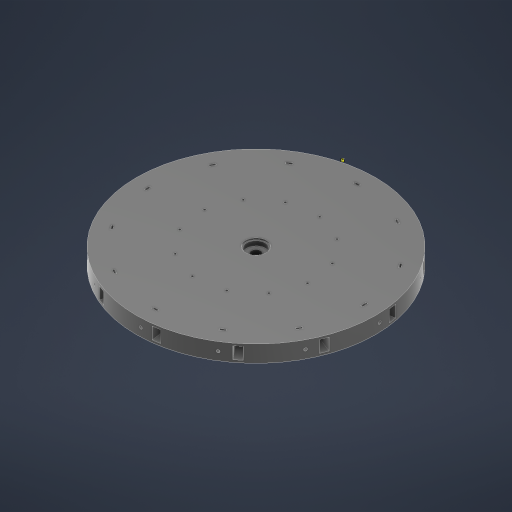
# Autodesk Inventor part: RotorBody
Saved by Autodesk Inventor 2023.1 (Build 271208000, 208)
## iProperties
Created: 2022-07-28
Part Number: RotorBody
Material: ABS Plastic
Document SubType Name: Modeling
Designer: ABL
Density: 1.06 g/cm^3
Appearance: Smooth - Black
Author: ABL
Autodesk Inventor part; units mm, degrees
ref_plane "YZ Plane" through (0, 0, 0) normal (1, 0, 0) x (0, 1, 0)
ref_plane "XZ Plane" through (0, 0, 0) normal (0, 1, 0) x (-1, 0, 0)
ref_plane "XY Plane" through (0, 0, 0) normal (0, 0, 1) x (1, 0, 0)
sketch "Sketch2" plane through (0, 0, 0) normal (0, 1, 0) x (-1, 0, 0)
  circle A0 centre (0, 0) radius 101.1611
  circle A1 centre (0, 0) radius 4.2
  dimension "d4" = 202.3223
  dimension "d101" = 8.4
  constraints: 2 centre point, 2 coincident
  measures "d4" diameter of A0
  measures "d101" diameter of A1
extrude "Extrusion1" add sketch "Sketch2" along normal blind 14.1
ref_plane "Work Plane4" through (-26.1824, 0, -97.7141) normal (-0.258819, 0, -0.9659258) x (0, -1, 0)
sketch "Sketch13" plane through (-27.2565, 0, -101.7227) normal (-0.258819, 0, -0.9659258) x (0, -1, 0)
  line L0 (-14.1, 101.1611) -> (-14.1, -101.1611) construction
  line L1 (0, 0) -> (-14.1, 0) construction
  line L2 (0, 0.05) -> (-14.1, 0.05)
  line L3 (-14.1, 0.05) -> (-14.1, -0.05)
  line L4 (-14.1, -0.05) -> (0, -0.05)
  line L5 (0, -0.05) -> (0, 0.05)
  line L6 (0, 0.05) -> (-14.1, -0.05) construction
  line L7 (-14.1, 0.05) -> (0, -0.05) construction
  point P0 (-7.05, 0)
  dimension "d136" = 0.1
  dimension "d139" = 7.05
  dimension "d140" = 2.05
  dimension "d141" = 4.2
  dimension "d142" = 3.8
  dimension "d146" = 4.1
  dimension "d147" = 4.3
  dimension "d153" = 4.2
  constraints: 8 end point, 2 parallel, 1 horizontal, 1 perpendicular
  measures "d153" distance of L2.end L3.end
sketch "Sketch10" plane through (0, 0, 0) normal (0, -1, 0) x (1, 0, 0)
  line L0 (0, 0) -> (-27.2565, -101.7227)
  line L1 (0, 0) -> (105.3111, 0) construction
  arc A0 (-27.2565, -101.7227) -> (30.0421, -100.9352) centre (0, 0) ccw
  line L2 (0, 0) -> (30.0421, -100.9352)
  line L3 (0, 0) -> (-27.2565, -101.7227) construction
  dimension "d96" = 105.3111
  dimension "d97" = 105
  dimension "d98" = 31.575
  constraints: 8 end point, 2 point on circle, 1 centre point, 1 coincident, 1 equal length, 1 horizontal
  measures "d96" distance of L0.start L0.end
  measures "d97" angle of L0 L1
  measures "d98" angle of L3 L2
sketch "Sketch8" plane through (0, 0, 0) normal (0, 1, 0) x (-1, 0, 0)
  circle A0 centre (0, 0) radius 105.3111
  circle A1 centre (0, 0) radius 101.2111
  circle A2 centre (0, 0) radius 4.2 projected
  line L0 (0, 0) -> (74.4662, -74.4662)
  line L1 (0, 0) -> (-101.7227, -27.2565)
  line L2 (0, 0) -> (0, -105.3111) construction
  point P0 (-97.7624, -26.1954)
  point P1 (71.5671, -71.5671)
  dimension "d81" = 210.6223
  dimension "d82" = 202.4223
  dimension "d184" = 120
  dimension "d185" = 45
  constraints: 6 end point, 3 point on circle, 2 centre point, 2 coincident, 1 vertical
  measures "d81" diameter of A0
  measures "d82" diameter of A1
  measures "d184" angle of L0 L1
  measures "d185" angle of L0 L2
extrude "Extrusion2" add sketch "Sketch8" along normal blind 14.1 separate body contours L1 A1 L0 A0 picked at (-26.5065, -98.9237)
pattern_circular "Circular Pattern5" [suppressed]
sketch "Sketch1" plane through (0, 0, 0) normal (0, 1, 0) x (-1, 0, 0)
  circle A0 centre (0, 0) radius 38.9611 construction
  arc A1 (-26.1824, -97.7141) -> (26.1824, -97.7141) centre (0, 0) ccw
  line L0 (0, 0) -> (26.1824, -97.7141)
  line L1 (0, 0) -> (101.1611, 0) construction
  line L2 (0, 0) -> (-26.1824, -97.7141)
  line L3 (26.1824, -97.7141) -> (10.0839, -37.6336)
  line L4 (-26.1824, -97.7141) -> (-10.0839, -37.6336)
  line L5 (-9.1645, -38.1966) -> (0.9762, -39.2945)
  line L6 (0.9762, -39.2945) -> (-5.5033, -99.1448)
  line L7 (-5.5033, -99.1448) -> (-15.6441, -98.0469)
  line L8 (-15.6441, -98.0469) -> (-9.1645, -38.1966)
  line L9 (0, 0) -> (0, -101.1611) construction
  line L10 (9.0759, -38.0159) -> (2.9502, -38.9728)
  line L11 (2.9502, -38.9728) -> (12.2411, -98.4515)
  line L12 (12.2411, -98.4515) -> (18.3668, -97.4946)
  line L13 (18.3668, -97.4946) -> (9.0759, -38.0159)
  line L14 (-4.0942, -38.7455) -> (0, 0) construction
  circle A2 centre (-2.0471, -19.3727) radius 2.6
  circle A3 centre (0, 0) radius 101.1611 construction
  line L15 (5.3197, -87.5773) -> (0.9224, -87.7339)
  line L16 (0.9224, -87.7339) -> (0.9794, -89.3329)
  line L17 (0.9794, -89.3329) -> (5.3766, -89.1763)
  line L18 (5.3766, -89.1763) -> (5.3197, -87.5773)
  line L19 (0, 0) -> (3.121, -87.6556) construction
  line L20 (0.9224, -87.7339) -> (-4.2078, -87.1785) construction
  line L21 (5.3197, -87.5773) -> (10.4181, -86.7809) construction
  line L22 (3.178, -89.2546) -> (3.5996, -101.0971) construction
  line L23 (-4.0942, -38.7455) -> (-5.145, -48.6902) construction
  line L24 (5.3481, -88.3768) -> (0.9509, -88.5334) construction
  point P0 (6.013, -38.4943)
  point P1 (3.1495, -88.4551)
  point P2 (-4.0942, -38.7455)
  dimension "d0" = 77.9223
  dimension "d1" = 101.1611
  dimension "d2" = 75
  dimension "d3" = 30
  dimension "d7" = 10.2
  dimension "d8" = 60.2
  dimension "d9" = 6.2
  dimension "d10" = 60.2
  dimension "d11" = 2
  dimension "d15" = 1.0781
  dimension "d16" = 1.0781
  dimension "d17" = 5.2
  dimension "d66" = 4.4
  dimension "d67" = 1.6
  dimension "d79" = 90
  dimension "d80" = 11.85
  dimension "d108" = 19.4806
  dimension "d122" = 10
  dimension "d189" = 10.2654
  dimension "d190" = 7.4925
  dimension "d191" = 17.7579
  constraints: 50 end point, 8 midpoint, 7 perpendicular, 7 point on circle, 6 point on line, 4 parallel, 3 centre point, 3 coincident, 2 collinear, 2 equal length, 2 tangent, 1 horizontal
  measures "d0" diameter of A0
  measures "d1" radius of A1
  measures "d2" angle of L0 L1
  measures "d3" angle of L2 L0
  measures "d7" distance of L6.end L7.end
  measures "d8" distance of L5.end L6.end
  measures "d9" distance of L12.end L11.end
  measures "d10" distance of L11.end L10.end
  measures "d11" distance of L10.end L5.end
  measures "d15" distance of L5.start L4.end
  measures "d16" distance of L3.end L10.start
  measures "d17" diameter of A2
  measures "d66" distance of L15.start L15.end
  measures "d67" distance of L15.end L16.end
  measures "d79" angle of L19 L15
  measures "d80" distance of L22.start L22.end
  measures "d108" distance of A0.centre A2.centre
  measures "d122" distance of L14.start L23.end
  measures "d189" distance from line of L7.end L2
  measures "d190" distance from line of L0 L12.end
  measures "d191" distance of L11.end L6.end
extrude "driveMagnet_slot" cut sketch "Sketch1" along normal blind 10.1 contours L5 L6 L7 L8 bodies 1
extrude "halbachMagnet_slot" cut sketch "Sketch1" along normal blind 12.1 contours L13 L12 L11 L10 bodies 1
sketch "Sketch4" plane through (-12.2411, 0, -98.4515) normal (0.154334, 0, 0.9880187) x (0.9880187, 0, -0.154334)
  line L0 (0, 0) -> (0, 12.1) projected
  line L1 (0, 2) -> (-6.2, 2)
  line L2 (-6.2, 2) -> (-6.2, 12.2)
  line L3 (-6.2, 12.2) -> (0, 12.2)
  line L4 (0, 12.2) -> (0, 2)
  line L5 (0, 0) -> (-6.2, 0) projected
  point P0 (-3.1, 0)
  dimension "d31" = 6.2
  dimension "halbachMagnet_slotHeight" = 10.2
  dimension "d33" = 2
  constraints: 8 end point, 2 parallel, 1 horizontal, 1 perpendicular, 1 point on line
  measures "d31" distance of L2.end L3.end
  measures "halbachMagnet_slotHeight" distance of L1.end L2.end
  measures "d33" distance between parallel lines of L5 L1
extrude "halbachMagnet_opening" cut sketch "Sketch4" against normal through all bodies 1
extrude "halbachMagnet_roof" add sketch "Sketch1" along normal blind 2 contours L13 L12 L11 L10 bodies 1
extrude "halbachMagnet_slotTopSurfaceIndent" cut sketch "Sketch1" along normal blind 0.2 contours L13 L12 L11 L10 bodies 1
extrude "sensorMagnet_slot" cut sketch "Sketch1" along normal blind 2.7667 contours A2 bodies 1
extrude "rotorBandNut_slot" cut sketch "Sketch1" against normal blind 9.2 from surface at 14.1 contours L18 L17 L16 L15 bodies 1
hole "rotorBandNut_removalHole" at (-3.1495, 0, -88.4551) direction (0, 1, 0) diameter 1.4 depth 4.9 bodies 1
pattern_circular "Sketch1_Pattern" count 12 over 360 about axis through (0, -10, 0) along (0, 1, 0) of "rotorBandNut_removalHole", "rotorBandNut_slot", "sensorMagnet_slot", "halbachMagnet_roof", "halbachMagnet_opening", "halbachMagnet_slot", "driveMagnet_slot", "halbachMagnet_slotTopSurfaceIndent" bodies 1
sketch "Sketch7" plane through (-5.3197, 0, -87.5773) normal (-0.0355833, 0, -0.9993667) x (-0.9993667, 0, 0.0355833)
  line L0 (-2.2, 4.9) -> (-2.2, 7) construction
  line L1 (-4.4, 4.9) -> (0, 4.9) projected
  point P0 (-2.2, 0)
  dimension "d71" = 2.1
  constraints: 2 end point, 1 coincident, 1 midpoint, 1 vertical
  measures "d71" distance of L0.start L0.end
ref_plane "Work Plane2" through (-3.7473, 0, -105.2444) normal (0.0355833, 0, 0.9993667) x (0, 1, 0)
ref_plane "Work Plane1" through (-5.3197, 9.5, -87.5773) normal (0.0355833, 0, 0.9993667) x (0, 1, 0)
sketch "Sketch9" plane through (-3.7473, 0, -105.2444) normal (0.0355833, 0, 0.9993667) x (0, 1, 0)
  line L0 (0, 0) -> (7.05, 0) construction
  dimension "d85" = 7.05
  constraints: 2 coincident, 2 end point, 1 horizontal
  measures "d85" distance of L0.start L0.end
hole "rotorBandBolt_hole" at (-3.7473, 7.05, -105.2444) direction (0.0355833, 0, 0.9993667) diameter 2.4 depth 24 counterbore diameter 4.08 counterbore depth 2.1 bodies 2 1
sketch "Sketch18" plane through (-0.9224, 4.9, -87.7339) normal (-0.0355833, 0, -0.9993667) x (-0.9993667, 0, 0.0355833)
  line L0 (0, 0.8798) -> (0, 3.4202)
  line L1 (0, 3.4202) -> (2.2, 4.6903)
  line L2 (2.2, 4.6903) -> (4.4, 3.4202)
  line L3 (4.4, 3.4202) -> (4.4, 0.8798)
  line L4 (4.4, 0.8798) -> (2.2, -0.3903)
  line L5 (2.2, -0.3903) -> (0, 0.8798)
  circle A0 centre (2.2, 2.15) radius 1.2 projected
  line L6 (0, 9.2) -> (4.4, 9.2) projected
  line L7 (0, 9.2) -> (0, 0) projected
  line L8 (0, 0) -> (4.4, 0) projected
  line L9 (4.4, 0) -> (4.4, 9.2) projected
  point P0 (2.2, -4.9)
  point P1 (2.2, 2.15)
  dimension "d176" = 4.4
  constraints: 12 end point, 1 coincident, 1 vertical, 13 other
  measures "d176" distance between parallel lines of L3 L0
extrude "rotorBandNut_hexCutaway" cut sketch "Sketch18" along normal up to surface (1.6 mm away) contours L0 L1 L2 L3 L4 L8 L5 | L8 L4 L5 | A0 bodies 1
pattern_circular "BoltHoles" count 12 over 360 about axis through (0, -10, 0) along (0, 1, 0) of "rotorBandBolt_hole", "rotorBandNut_hexCutaway" bodies 1 2
sketch "Sketch11" plane through (0, 0, 0) normal (0, -1, 0) x (1, 0, 0)
  circle A0 centre (0, 0) radius 9
  circle A1 centre (0, 0) radius 8
  dimension "d102" = 18
  dimension "d105" = 16
  constraints: 2 centre point, 2 coincident
  measures "d102" diameter of A0
  measures "d105" diameter of A1
extrude "flangeBearing_flangeInset" cut sketch "Sketch11" against normal blind 1.4 bodies 1
extrude "flangeBearing_bodyInset" cut sketch "Sketch11" against normal blind 5.2 contours A1 bodies 1
ref_plane "Work Plane3" through (0, 7.05, 0) normal (0, -1, 0) x (1, 0, 0)
mirror "flangeBearing_mirror" about plane through (0, 7.05, 0) normal (0, -1, 0) of "flangeBearing_flangeInset", "flangeBearing_bodyInset" bodies 1
hole "halbachMagnet_removalHole" at (-6.013, 0, -38.4943) direction (0, 1, 0) diameter 2 depth 12.1 bodies 1
sketch "Sketch12" plane through (-9.0759, 2, -38.0159) normal (-0.154334, 0, -0.9880187) x (-0.9880187, 0, 0.154334)
  line L0 (-6.2, 0) -> (0, 0) projected
  line L1 (-3.1, 0) -> (-3.1, -2) construction
  line L2 (-3.1, -2) -> (-4.1, -2)
  line L3 (-4.1, -2) -> (-4.1, 0)
  line L4 (-4.1, 0) -> (-3.1, 0)
  line L5 (-3.1, -2) -> (-2.1, -2)
  line L6 (-2.1, -2) -> (-2.1, 0)
  line L7 (-2.1, 0) -> (-3.1, 0)
  point P0 (-2.1, 0)
  point P1 (-4.1, 0)
  dimension "d116" = 1
  constraints: 14 end point, 2 parallel, 2 symmetric about line, 1 midpoint, 1 perpendicular, 1 vertical
  measures "d116" distance of L1.end L2.end
extrude "halbachMagnet_removalChannel" cut sketch "Sketch12" along normal blind 10 bodies 1
hole "driveMagnet_removalHole" at (5.145, 0, -48.6902) direction (0, 1, 0) diameter 2 depth 14.1 bodies 1
pattern_circular "Circular Pattern3" count 12 over 360 about axis through (0, -10, 0) along (0, 1, 0) of "halbachMagnet_removalHole", "halbachMagnet_removalChannel", "driveMagnet_removalHole" bodies 1
sketch "Sketch17" plane through (0, 0, 0) normal (0, -1, 0) x (-0.9659258, 0, -0.258819)
  circle A0 centre (0, 0) radius 8 construction
  line L0 (0, 0) -> (27.2565, -101.7227) construction
  arc A1 (91.2021, 52.6556) -> (-91.2021, 52.6556) centre (0, 0) ccw construction
  line L1 (0, 0) -> (105.3111, 0) construction
  arc A2 (27.2565, -101.7227) -> (101.7227, -27.2565) centre (0, 0) ccw
  line L2 (0, 0) -> (101.7227, -27.2565)
  line L3 (0, 0) -> (27.2565, -101.7227) construction
  arc A3 (-74.4662, -74.4662) -> (27.2565, -101.7227) centre (0, 0) ccw
  line L4 (0, 0) -> (-74.4662, -74.4662)
  line L5 (0, 0) -> (27.2565, -101.7227) construction
  dimension "d154" = 75
  dimension "d155" = 60
  dimension "d156" = 60
  constraints: 12 end point, 7 point on circle, 2 centre point, 2 coincident, 2 concentric, 1 equal length, 1 horizontal
  measures "d154" angle of L0 L1
  measures "d155" angle of L3 L2
  measures "d156" angle of L4 L5
extrude "rotorBand_printingExport" [suppressed]
equation "\"d4\" = 2 * rotorRadius"
equation "\"d5\" = rotorThickness"
equation "\"d0\" = 2 * driveMagnet_centerSpacingRadius"
equation "\"d1\" = rotorRadius"
equation "\"d7\" = driveMagnet_width + 2 * gap"
equation "\"d8\" = driveMagnet_length + 2 * gap"
equation "\"d10\" = halbachMagnet_length + 2 * gap"
equation "\"d11\" = wallgap"
equation "\"d16\" = d15"
equation "\"d17\" = sensorMagnet_diameter + 2 * gap"
equation "\"d20\" = gap + halbachMagnet_width + wallgap"
equation "\"d33\" = wallgap"
equation "\"d36\" = wallgap"
equation "\"d22\" = sensorMagnet_height + gap"
equation "\"d68\" = 0.5 * rotorBandSquareNut_sideLength + 0.5 * halbachMagnet_slotHeight + wallgap + gap"
equation "\"d71\" = 0.5 * rotorBandSquareNut_sideLength + gap"
equation "\"gap\" = 0.1"
equation "\"airgap\" = 0.4"
equation "\"driveMagnet_height\" = 5"
equation "\"halbachMagnet_width\" = 10"
equation "\"halbachMagnet_height\" = 3"
equation "\"sensorMagnet_diameter\" = 5"
equation "\"sensorMagnet_height\" = 2.66667"
equation "\"wallgap\" = 2"
equation "\"driveMagnet_centerSpacingRadius\" = 38.96113"
equation "\"rotorThickness\" = 14.1"
equation "\"shaftDiameter\" = 8"
equation "\"flangeBearing_outerDiameter\" = 16"
equation "\"flangeBearing_innerDiameter\" = shaftDiameter"
equation "\"flangeBearing_height\" = 5"
equation "\"flangeBearing_flangeHeight\" = 1"
equation "\"flangeBearing_flangeDiameter\" = 18"
equation "\"statorThickness\" = 16"
equation "\"rotor_mountingLipHeight\" = 8"
equation "\"rotorRadius\" = 101.16113"
equation "\"rotorBandSquareNut_sideLength\" = 4"
equation "\"rotorBandHexNut_height\" = 1.2"
equation "\"rotorBandHexNut_sideToSide\" = 4"
equation "\"rotorBandSquareNut_height\" = 1.2"
equation "\"rotorBandBolt_headHeight\" = 2"
equation "\"rotorBandBolt_headDiameter\" = 3.98"
equation "\"rotorBandBolt_diameter\" = 2"
equation "\"rotorBandThickness\" = 4.1"
equation "\"flangeCoupling_collarOuterDiameter\" = 16"
equation "\"flangeCoupling_flangeHoleEdgeToEdge\" = 2.05"
equation "\"flangeCoupling_innerDiameter\" = 8"
equation "\"flangeCoupling_flangeHoleDiameter\" = 3.9"
equation "\"flangeCoupling_flangeHeight\" = 3.1"
equation "\"flangeCoupling_flangeDiameter\" = 32"
equation "\"flangeCoupling_height\" = 13.1"
equation "\"flangeCoupling_mountHoleDiameter\" = 3.9"
equation "\"flangeCoupling_mountHoleEdgeToEdge\" = 2.05"
equation "\"statorRadius\" = 99.16113"
equation "\"coilThickness\" = 12"
equation "\"statorMountBolt_diameter\" = 4"
equation "\"statorMountBolt_headDiameter\" = 7"
equation "\"statorMountBolt_headHeight\" = 4"
equation "\"statorMountBolt_shaftLength\" = 17.1"
equation "\"statorMountHexNut_height\" = 4"
equation "\"statorMountHexNut_sideToSide\" = 8"
equation "\"sensorMagnet_ringRadius\" = 23.48057"
equation "\"coil_percentCoverage\" = 0.6"
equation "\"statorSpokeDegrees\" = 4deg"
equation "\"coil_bulge\" = 3"
equation "\"statorCoilBolt_shaftLength\" = 19.3"
equation "\"statorCoilHexNut_height\" = 1.2"
equation "\"statorCoilBolt_headHeight\" = 2"
equation "\"statorCoilBolt_diameter\" = 2"
equation "\"statorCoilBolt_headDiameter\" = 3.98"
equation "\"statorCoilHexNut_sideToSide\" = 4"
equation "\"magnetWire_outerDiameter\" = 0.8128"
equation "\"printingLayerHeight\" = 0.2"
equation "\"circuitBoard_height\" = 1.6"
equation "\"hallEffectSensor_width\" = 1.6"
equation "\"hallEffectSensor_length\" = 3"
equation "\"hallEffectSensor_height\" = 1.1"
equation "\"hallEffectSensor_pinLength\" = 0.6"
equation "\"circuitboardMountHexNut_height\" = 1.2"
equation "\"circuitboardMountHexNut_sideToSide\" = 4"
equation "\"circuitboardMountBolt_headHeight\" = 2"
equation "\"circuitboardMountBolt_shaftLength\" = 12"
equation "\"circuitboardMountBolt_diameter\" = 2"
equation "\"circuitboardMountBolt_headDiameter\" = 3.98"
equation "\"statorShellBolt_headDiameter\" = 5.68"
equation "\"statorShellHexNut_height\" = 2.3"
equation "\"statorShellBolt_shaftLength\" = 12.6"
equation "\"statorShellBolt_headHeight\" = 3"
equation "\"statorShellHexNut_sideToSide\" = 5.3"
equation "\"statorShellBolt_diameter\" = 3"
equation "\"statorShellBolt_countersinkDepth\" = 3.4"
equation "\"flangeCoupling_mountHoleCenterToCouplingCenter\" = 12"
equation "\"driveMagnet_width\" = 10"
equation "\"driveMagnet_length\" = 60"
equation "\"halbachMagnet_length\" = 60"
